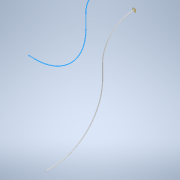
# Autodesk Inventor part: Cable 220V - 2.5in - 1.5m
Saved by Autodesk Inventor 2020.3 (Build 243373000, 373)
## iProperties
Created: 2020-07-06
Part Number: Cable 220V - 2.5in - 1.5m
Material: Acetal Resin, Black
Document SubType Name: Modeling
Designer: Bruno
Density: 1.425 g/cm^3
Appearance: Smooth - Black
Author: Bruno
Autodesk Inventor part; units mm, degrees
ref_plane "YZ Plane" through (0, 0, 0) normal (1, 0, 0) x (0, 1, 0)
ref_plane "XZ Plane" through (0, 0, 0) normal (0, 1, 0) x (-1, 0, 0)
ref_plane "XY Plane" through (0, 0, 0) normal (0, 0, 1) x (1, 0, 0)
ref_plane "Work Plane1" through (0, 0, 0) normal (0, -0.0021, 1) x (1, 0, 0)
ref_plane "Work Plane3" through (0, 0, 0) normal (0, 0, 1) x (1, 0, 0)
sketch "Sketch2" plane through (0, 0, 0) normal (0, 0, 1) x (1, 0, 0)
  circle A0 centre (0, 0) radius 3.175
  dimension "d13" = 6.35
  constraints: 1 centre point, 1 coincident
  measures "d13" diameter of A0
sketch3d "3D Sketch1"
  line L0 (0, 0, 0) -> (0, -0.0209, 10)
  arc A0 (0, -0.0209, 10) -> (0, -240.5217, 249.4982) centre (0, -240.0204, 9.4987) ccw
  line L1 (0, -240.5217, 249.4982) -> (0, -349.6851, 249.2702)
  arc A1 (0, -349.6851, 249.2702) -> (0, -750.5205, 649.2693) centre (0, -350.5205, 649.2693) ccw
  line L2 (0, -750.5205, 649.2693) -> (0, -750.5205, 698.4329)
  dimension "d0" = 250
  dimension "d1" = 750
  dimension "d2" = 90
  dimension "d6" = 450
  dimension "d7" = 0
  dimension "d9" = 240
  dimension "d10" = 400
sweep "Sweep2" add profiles "Sketch2" path "3D Sketch1"
body "Solid2"
